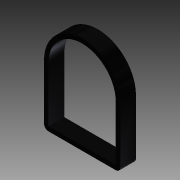
# Autodesk Inventor part: ZIP TIE Y BEARINGS
Saved by Autodesk Inventor 2013 (Build 170138000, 138)
## iProperties
Created: 2014-06-22
Part Number: ZIP TIE Y BEARINGS
Material: Generic
Document SubType Name: Modeling
Designer: employee
Density: 1 g/cm^3
Author: employee
Autodesk Inventor part; units mm, degrees
ref_plane "YZ Plane" through (0, 0, 0) normal (1, 0, 0) x (0, 1, 0)
ref_plane "XZ Plane" through (0, 0, 0) normal (0, 1, 0) x (-1, 0, 0)
ref_plane "XY Plane" through (0, 0, 0) normal (0, 0, 1) x (1, 0, 0)
sketch "Sketch1" plane through (0, 0, 0) normal (0, 0, 1) x (1, 0, 0)
  line L0 (0, -5.715) -> (1.5, -5.715) construction
  line L1 (1.5, 0) -> (1.5, -5.715) construction
  line L2 (1.5, 0) -> (0, 0) construction
  line L3 (0, 0) -> (0, -5.715) construction
  circle A0 centre (9, 6.4952) radius 4 construction
  circle A1 centre (9, 6.4952) radius 7.5 construction
  line L4 (16.5, -5.715) -> (18, -5.715) construction
  line L5 (18, 0) -> (18, -5.715) construction
  line L6 (18, 0) -> (16.5, 0) construction
  line L7 (16.5, 0) -> (16.5, -5.715) construction
  line L8 (1.5, -5.715) -> (16.5, -5.715)
  line L9 (16.5, -5.715) -> (16.5, 6.4952)
  arc A2 (16.5, 6.4952) -> (1.5, 6.4952) centre (9, 6.4952) ccw
  line L10 (1.5, -5.715) -> (1.5, 6.4952)
  arc A3 (17.5, 6.4952) -> (0.5, 6.4952) centre (9, 6.4952) ccw
  line L11 (17.5, 6.4952) -> (17.5, -6.715)
  line L12 (17.5, -6.715) -> (0.5, -6.715)
  line L13 (0.5, -6.715) -> (0.5, 6.4952)
  dimension "d0" = 1
  constraints: 12 end point, 6 point on circle, 4 tangent, 2 centre point, 2 parallel, 1 concentric, 1 perpendicular, 3 other
  measures "d0" radial gap between concentric circles of A3 A1
extrude "Extrusion1" add sketch "Sketch1" along normal blind 3.5
fillet "Fillet1" radius 1 2 edges at (17.5, -6.715, 1.75) (0.5, -6.715, 1.75)
body "Solid1"
